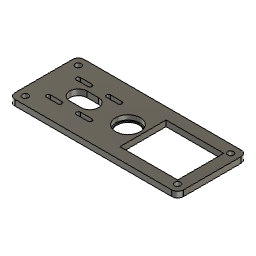
body-plate (Autodesk Fusion 360 design; units mm, degrees)
Autodesk Fusion 360 part; units mm, degrees
sketch "Sketch1" plane through (0, 0, 0) normal (0, 0, 1) x (1, 0, 0)
  circle A0 centre (0, 0) radius 10.6
  line L0 (-33, 7.5) -> (-43, 7.5)
  arc A1 (-43, 7.5) -> (-43, -7.5) centre (-43, 0) ccw
  line L1 (-43, -7.5) -> (-33, -7.5)
  arc A2 (-33, -7.5) -> (-33, 7.5) centre (-33, 0) ccw
  line L2 (-25.5, 0) -> (-50.5, 0) construction
  line L3 (-20, 14.75) -> (-30, 14.75)
  arc A3 (-30, 14.75) -> (-30, 11.25) centre (-30, 13) ccw
  line L4 (-30, 11.25) -> (-20, 11.25)
  arc A4 (-20, 11.25) -> (-20, 14.75) centre (-20, 13) ccw
  line L5 (-18.25, 13) -> (-31.75, 13) construction
  line L6 (-43, 0) -> (-33, 0) construction
  line L7 (-30, 13) -> (-20, 13) construction
  line L8 (0, 0) -> (-73, 0) construction
  line L9 (-20, -14.75) -> (-30, -14.75)
  arc A5 (-30, -11.25) -> (-30, -14.75) centre (-30, -13) ccw
  line L10 (-30, -11.25) -> (-20, -11.25)
  arc A6 (-20, -14.75) -> (-20, -11.25) centre (-20, -13) ccw
  line L11 (-38, 0) -> (-38, 13) construction
  line L12 (-56, 14.75) -> (-46, 14.75)
  arc A7 (-46, 11.25) -> (-46, 14.75) centre (-46, 13) ccw
  line L13 (-46, 11.25) -> (-56, 11.25)
  arc A8 (-56, 14.75) -> (-56, 11.25) centre (-56, 13) ccw
  line L14 (-56, -14.75) -> (-46, -14.75)
  arc A9 (-56, -11.25) -> (-56, -14.75) centre (-56, -13) ccw
  line L15 (-46, -11.25) -> (-56, -11.25)
  arc A10 (-46, -14.75) -> (-46, -11.25) centre (-46, -13) ccw
  line L16 (-73, 30) -> (73, 30)
  line L17 (73, 30) -> (73, -30)
  line L18 (73, -30) -> (-73, -30)
  line L19 (-73, -30) -> (-73, 30)
  line L20 (-63, 20) -> (-13, 20) construction
  line L21 (-13, 20) -> (-13, -20) construction
  line L22 (-13, -20) -> (-63, -20) construction
  line L23 (-63, -20) -> (-63, 20) construction
  line L24 (0, 30) -> (0, -30) construction
  line L25 (63, 20) -> (13, 20)
  line L26 (63, -20) -> (63, 20)
  line L27 (13, -20) -> (63, -20)
  line L28 (13, 20) -> (13, -20)
  circle A11 centre (-66, 23) radius 2.6
  circle A12 centre (-66, -23) radius 2.6
  circle A13 centre (66, 23) radius 2.6
  circle A14 centre (66, -23) radius 2.6
  point P0 (-38, 0)
  point P1 (0, -30)
  point P2 (-63, 0)
  dimension "d1" = 21.2
  dimension "d2" = 10
  dimension "d3" = 15
  dimension "d4" = 20
  dimension "d5" = 26
  dimension "d6" = 3.5
  dimension "d7" = 26
  dimension "d12" = 7
  dimension "d13" = 7
  dimension "d14" = 7
  dimension "d15" = 10
  dimension "d16" = 10
  dimension "d17" = 5.2
  dimension "d18" = 7
  dimension "d19" = 7
  constraint coincident A0.centre L8.start
  constraint tangent L0 A1
  constraint tangent A1 L1
  constraint parallel L0 L1
  constraint tangent L1 A2
  constraint tangent L0 A2
  constraint midpoint A2 L2.start
  constraint midpoint A1 L2.end
  constraint horizontal L2
  constraint tangent L3 A3
  constraint tangent A3 L4
  constraint parallel L3 L4
  constraint tangent L4 A4
  constraint tangent L3 A4
  constraint midpoint A4 L5.start
  constraint midpoint A3 L5.end
  constraint horizontal L5
  constraint coincident A1.centre L6.start
  constraint coincident A2.centre L6.end
  constraint coincident A3.centre L7.start
  constraint coincident A4.centre L7.end
  constraint equal L6 L7
  constraint parallel L2 L8
  constraint symmetric L3.start L8 L9.start
  constraint symmetric L3.end L8 L9.end
  constraint symmetric A3.end L8 A5.start
  constraint symmetric L4.end L8 L10.end
  constraint symmetric A3 L8 A5
  constraint symmetric A4 L8 A6
  constraint midpoint L6 P0
  constraint coincident P0 L11.start
  constraint perpendicular L8 L11
  constraint symmetric L3.start L11 L12.start
  constraint symmetric L3.end L11 L12.end
  constraint symmetric A3.end L11 A7.start
  constraint symmetric L4.end L11 L13.end
  constraint symmetric A3 L11 A7
  constraint symmetric A4 L11 A8
  constraint symmetric L8 L12.start L14.start
  constraint symmetric L8 L12.end L14.end
  constraint symmetric L8 A7.start L15.start
  constraint symmetric L8 A7 A10
  constraint symmetric L8 L13.end A9.start
  constraint symmetric L8 A8 A9
  constraint horizontal L16
  constraint vertical L17
  constraint horizontal L18
  constraint vertical L19
  constraint midpoint L8.end L19
  constraint midpoint L18 P1
  constraint vertical A0.centre P1
  constraint horizontal L20
  constraint vertical L21
  constraint horizontal L22
  constraint vertical L23
  constraint midpoint L23 P2
  constraint horizontal A0.centre P2
  constraint midpoint L16 L24.start
  constraint coincident P1 L24.end
  constraint symmetric L20.start L24 L25.start
  constraint symmetric L20.end L24 L25.end
  constraint symmetric L21.end L24 L27.start
  constraint symmetric L22.end L24 L26.start
  constraint symmetric L8 A11 A12
  constraint symmetric L24 A11 A13
  constraint symmetric L24 A12 A14
  measures "d1" diameter of A0
  measures "d2" distance of A2.centre A1.centre
  measures "d3" distance of L0 L1
  measures "d4" horizontal distance of A0.centre A4.centre
  measures "d5" distance of A4.centre A6.centre
  measures "d6" distance of L3 L4
  measures "d7" distance of A4.centre A7.centre
  measures "d12" distance of A8.centre L23
  measures "d13" distance of A8.centre L20
  measures "d14" distance of A4.centre L21
  measures "d15" distance of L19 L23
  measures "d16" distance of L16 L20
  measures "d17" diameter of A11
  measures "d18" distance of L19 A11.centre
  measures "d19" distance of L16 A11.centre
extrude "Extrude1" add sketch "Sketch1" along normal blind 5
sketch "Sketch2" plane through (0, 0, 0) normal (0, 0, 1) x (1, 0, 0)
  circle A0 centre (0, 0) radius 11
  circle A1 centre (0, 0) radius 9.5
  dimension "d22" = 19
  dimension "d23" = 22
  constraint coincident A0.centre A1.centre
  measures "d22" diameter of A1
  measures "d23" diameter of A0
extrude "Extrude2" add sketch "Sketch2" along normal blind 1
fillet "Fillet1" radius 5 4 edges at (-73, 30, 2.5) (-73, -30, 2.5) (73, 30, 2.5) (73, -30, 2.5)
